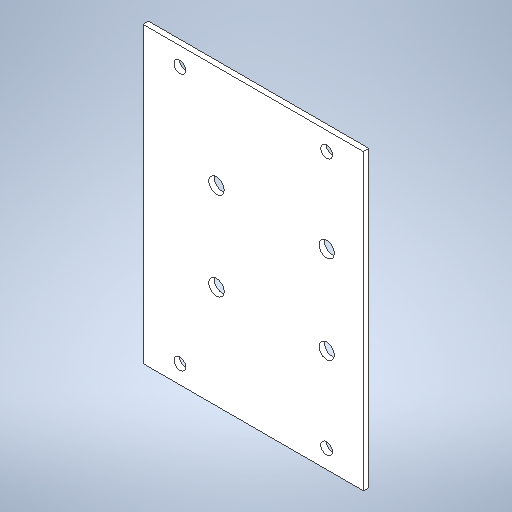
# Autodesk Inventor part: キャスター土台
Saved by Autodesk Inventor 2026.2 (Build 302298010, 298A)
## iProperties
Created: 2026-05-06
Part Number: キャスター土台
Material: 一般
Document SubType Name: Modeling
Designer: Yagis
Density: 1 g/cm^3
Appearance: 既定
Author: Yagis
Autodesk Inventor part; units mm, degrees
ref_plane "YZ Plane" through (0, 0, 0) normal (1, 0, 0) x (0, 1, 0)
ref_plane "XZ Plane" through (0, 0, 0) normal (0, 1, 0) x (-1, 0, 0)
ref_plane "XY Plane" through (0, 0, 0) normal (0, 0, 1) x (1, 0, 0)
sketch "スケッチ1" plane through (0, 0, 0) normal (0, 0, 1) x (1, 0, 0)
  line L0 (0, 0) -> (60, 0)
  line L1 (60, 0) -> (60, 80)
  line L2 (60, 80) -> (0, 80)
  line L3 (0, 80) -> (0, 0)
  dimension "d0" = 80
  dimension "d1" = 60
  constraints: 8 end point, 2 parallel, 1 horizontal, 1 perpendicular
  measures "d0" distance of L0.end L1.end
  measures "d1" distance of L1.end L2.end
extrude "押し出し1" add sketch "スケッチ1" along normal blind 1.5
sketch "スケッチ2" plane through (0, 0, 1.5) normal (0, 0, 1) x (1, 0, 0)
  line L0 (60, 0) -> (60, 80) projected
  line L1 (0, 0) -> (60, 0) projected
  line L2 (60, 80) -> (0, 80) projected
  point P0 (10, 5)
  point P1 (50, 5)
  point P2 (50, 75)
  point P3 (10, 75)
  dimension "d4" = 10
  dimension "d5" = 40
  dimension "d7" = 5
  dimension "d8" = 5
  constraints: 2 horizontal alignment, 2 vertical alignment
  measures "d4" distance from line of L0 point (50, 5)
  measures "d5" distance of point (10, 5) point (50, 5)
  measures "d7" distance from line of L1 point (50, 5)
  measures "d8" distance from line of point (50, 75) L2
hole "穴1" at (10, 5, 1.5) at (50, 5, 1.5) at (50, 75, 1.5) at (10, 75, 1.5) direction (0, 0, -1) diameter 3.2 depth 8.8 tip angle 118
sketch "スケッチ3" plane through (0, 0, 1.5) normal (0, 0, 1) x (1, 0, 0)
  line L0 (60, 80) -> (0, 80) projected
  line L1 (60, 0) -> (60, 80) projected
  point P0 (0, 0)
  point P1 (20, 52)
  point P2 (50, 52)
  point P3 (50, 28)
  point P4 (20, 28)
  dimension "d16" = 30
  dimension "d17" = 24
  dimension "d18" = 28
  dimension "d19" = 10
  constraints: 2 horizontal alignment, 2 vertical alignment
  measures "d16" distance of point (20, 52) point (50, 52)
  measures "d17" distance of point (50, 28) point (50, 52)
  measures "d18" distance from line of L0 point (50, 52)
  measures "d19" distance from line of L1 point (50, 52)
hole "穴2" at (20, 52, 1.5) at (50, 52, 1.5) at (50, 28, 1.5) at (20, 28, 1.5) direction (0, 0, -1) diameter 4.2 depth 8.8 tip angle 118
